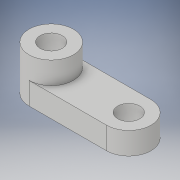
# Autodesk Inventor part: Part10
Saved by Autodesk Inventor 2017 (Build 210142000, 142)
## iProperties
Created: 2016-11-07
Part Number: Part10
Material: Generic
Document SubType Name: Modeling
Designer: s411888
Density: 1 g/cm^3
Appearance: Default
Author: s411888
Autodesk Inventor part; units mm, degrees
ref_plane "YZ Plane" through (0, 0, 0) normal (1, 0, 0) x (0, 1, 0)
ref_plane "XZ Plane" through (0, 0, 0) normal (0, 1, 0) x (-1, 0, 0)
ref_plane "XY Plane" through (0, 0, 0) normal (0, 0, 1) x (1, 0, 0)
sketch "Sketch1" plane through (0, 0, 0) normal (0, 1, 0) x (-1, 0, 0)
  line L0 (22.5427, 11.7774) -> (-21.9073, 11.7774)
  line L1 (-21.9073, 11.7774) -> (-21.9073, -13.6226)
  line L2 (-21.9073, -13.6226) -> (22.5427, -13.6226)
  line L3 (22.5427, -13.6226) -> (22.5427, 11.7774)
  circle A0 centre (-21.9073, -0.9226) radius 12.7
  circle A1 centre (-21.9073, -0.9226) radius 6.35
  circle A2 centre (22.5427, -0.9226) radius 12.7
  circle A3 centre (22.5427, -0.9226) radius 6.35
  point P0 (0, 0)
  dimension "d0" = 44.45
  dimension "d1" = 25.4
  dimension "d5" = 12.7
  dimension "d8" = 25.4
  dimension "d9" = 12.7
  constraints: 8 end point, 4 centre point, 2 coincident, 2 midpoint, 2 parallel, 1 horizontal, 1 perpendicular
  measures "d0" distance of L2.end L1.end
  measures "d1" distance of L1.end L0.end
  measures "d5" diameter of A1
  measures "d8" diameter of A2
  measures "d9" diameter of A3
extrude "Extrusion2" add sketch "Sketch1" along normal blind 12.7 contours A2 L2 A0 L0 | L3 A3 A2 | A0 L1 A1 | L3 A3 | A1 L1 picked at (21.023, -11.3214) picked at (-14.3032, 6.3463) picked at (19.6489, 0.8427) picked at (-19.8437, -0.4516)
extrude "Extrusion3" add sketch "Sketch1" along normal blind 12.7 contours A0 L1 A1 | L1 A1 A0
extrude "Extrusion4" cut sketch "Sketch1" along normal blind 12.7 contours A1 L1 | L1 A1
extrude "Extrusion5" add sketch "Sketch1" along normal blind 25.4 contours A2 L3 A3 | L3 A3 A2
extrude "Extrusion6" cut sketch "Sketch1" against normal blind 25.4 contours A3 L3 | L3 A3
extrude "Extrusion7" cut sketch "Sketch1" along normal blind 25.4 contours A3 L3 | L3 A3
body "Solid2"
